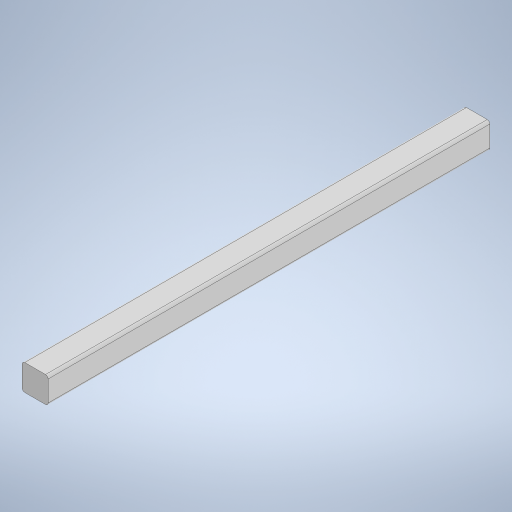
# Autodesk Inventor part: item40x40_1000
Saved by Autodesk Inventor 2024.4 (Build 284460000, 460)
## iProperties
Created: 2025-11-05
Part Number: item40x40_1000
Material: Generic
Document SubType Name: Modeling
Designer: jonas
Density: 1 g/cm^3
Appearance: Default
Author: jonas
Autodesk Inventor part; units mm, degrees
ref_plane "YZ Plane" through (0, 0, 0) normal (1, 0, 0) x (0, 1, 0)
ref_plane "XZ Plane" through (0, 0, 0) normal (0, 1, 0) x (-1, 0, 0)
ref_plane "XY Plane" through (0, 0, 0) normal (0, 0, 1) x (1, 0, 0)
sketch "Sketch1" plane through (0, 0, 0) normal (0, 1, 0) x (-1, 0, 0)
  line L0 (0, 12.4728) -> (0, -12.4728) construction
  line L1 (2.135, 0) -> (-2.135, 0) construction
  line L2 (16, 20) -> (-16, 20)
  line L3 (-20, 16) -> (-20, -16)
  line L4 (-16, -20) -> (16, -20)
  line L5 (20, -16) -> (20, 16)
  arc A0 (-16, 20) -> (-20, 16) centre (-16, 16) ccw
  arc A1 (-20, -16) -> (-16, -20) centre (-16, -16) ccw
  arc A2 (16, -20) -> (20, -16) centre (16, -16) ccw
  arc A3 (20, 16) -> (16, 20) centre (16, 16) ccw
  point P0 (0, 0)
  point P1 (0, 0)
  dimension "d1" = 4
  dimension "d2" = 4
  dimension "d3" = 40
  constraints: 12 end point, 8 point on circle, 8 tangent, 4 centre point, 2 equal radius, 2 horizontal, 2 midpoint, 2 parallel, 2 perpendicular, 1 coincident, 1 vertical, 2 other
  measures "d1" radius of A0
  measures "d2" radius of A2
  measures "d3" distance between parallel lines of L2 L4
extrude "Extrusion1" add sketch "Sketch1" along normal blind 680
body "Solid1"
